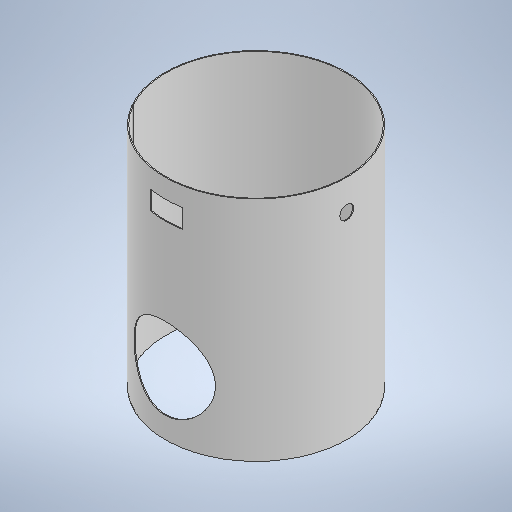
# Autodesk Inventor part: PRS 000 Filter1200 MAIN Shell
Saved by Autodesk Inventor 2026.2 (Build 302298000, 298)
## iProperties
Created: 2025-02-11
Part Number: PRS 000 Filter1200 MAIN Shell
Material: Steel
Document SubType Name: Sheet Metal
Designer: pokla
Mass: 197479 g
Surface Area: 84554.1 cm^2
Volume: 25156.5 cm^3
Density: 7.85 g/cm^3
Flat Pattern Width: 150 cm
Flat Pattern Length: 374.776 cm
Flat Pattern Area: 56216.4 cm^2
Sheet Metal Rule: Default_mm
Sheet Metal Width: 1500,000 mm
Sheet Metal Length: 3747,758 mm
Sheet Metal Area: 5621637,523 mm^2
Appearance: Default
Author: pokla
Autodesk Inventor part; units mm, degrees
sketch "Sketch13" plane through (0, 0, 0) normal (0, 0, 1) x (1, 0, 0)
  circle A0 centre (0, 0) radius 600 construction
  line L0 (0, 0) -> (0, -600)
  line L1 (0, 0) -> (-519.6152, -300)
  line L2 (0, 0) -> (600, 0)
  line L3 (0, 0) -> (0, -600)
  line L4 (0, 0) -> (0, -600)
  line L5 (0, 0) -> (534.6039, 272.3943)
  line L6 (0, 0) -> (0, 600)
  dimension "d53" = 1200
  dimension "d55" = 0
  dimension "d98" = 180
  dimension "d99" = 240
  dimension "d100" = 63
  dimension "d101" = 90
  constraints: 14 end point, 1 coincident, 1 point on line, 1 vertical, 9 other
  measures "d55" distance between parallel lines of L0 L4
  measures "d98" angle of L3 L6
  measures "d100" angle of L6 L5
  measures "d101" angle of L2 L6
ref_plane "WeldJoint" through (0, 0, -10) normal (0.5, -0.866, 0) x (0, 0, 1)
ref_plane "Inlet_Clock_Angle_plane" through (0, 0, -10) normal (0, 1, 0) x (0, 0, 1)
ref_plane "Charging" through (0, 0, -10) normal (1, 0, 0) x (0, 0, 1)
ref_plane "Accsess" through (0, 0, -10) normal (1, 0, 0) x (0, 0, 1)
sketch "Sketch14" plane through (0, 0, -10) normal (0.5, -0.866, 0) x (0, 0, 1)
  line L0 (1510, 594) -> (10, 594)
  line L1 (10, 594) -> (10, 600)
  line L2 (10, 600) -> (1510, 600)
  line L3 (1510, 600) -> (1510, 594)
  line L4 (10, 0) -> (1510, 0)
  line L5 (10, 600) -> (-20, 600) construction
  line L6 (10, 594) -> (-20, 594) construction
  arc A0 (-20, 594) -> (-109.2789, 539.0476) centre (-20, 494) ccw construction
  arc A1 (-109.2789, 539.0476) -> (-234, 15) centre (929.3202, 15) ccw construction
  line L7 (-234, 15) -> (-234, 0) construction
  line L8 (10, 0) -> (-234, 0) construction
  arc A2 (-20, 600) -> (-114.6356, 541.7504) centre (-20, 494) ccw construction
  arc A3 (-114.6356, 541.7504) -> (-240, 15) centre (929.3202, 15) ccw construction
  line L9 (-240, 15) -> (-240, 0) construction
  line L10 (-234, 0) -> (-240, 0) construction
  line L11 (1510, 594) -> (1540, 594)
  line L12 (1510, 600) -> (1540, 600)
  line L13 (1510, 0) -> (1754, 0) construction
  line L14 (1760, 0) -> (1760, 15) construction
  arc A4 (1760, 15) -> (1634.6356, 541.7504) centre (590.6798, 15) ccw construction
  arc A5 (1634.6356, 541.7504) -> (1540, 600) centre (1540, 494) ccw construction
  line L15 (1754, 0) -> (1754, 15) construction
  line L16 (1754, 0) -> (1760, 0) construction
  arc A6 (1754, 15) -> (1629.2789, 539.0476) centre (590.6798, 15) ccw construction
  arc A7 (1629.2789, 539.0476) -> (1540, 594) centre (1540, 494) ccw construction
  line L17 (-156.8588, 530) -> (-610, 530)
  line L18 (-610, 530) -> (-610, 450)
  line L19 (-610, 450) -> (-156.8588, 450)
  line L20 (-156.8588, 450) -> (-156.8588, 530)
  line L21 (1760, 15) -> (1790, 15) construction
  line L22 (1790, 15) -> (1790, 0) construction
  line L23 (1790, 0) -> (1760, 0) construction
  line L24 (-610, 610) -> (-610, 530)
  line L25 (-610, 610) -> (-604, 610)
  line L26 (-604, 610) -> (-604, 530)
  line L27 (-115.4356, 543.7196) -> (-164.9441, 431.7071)
  line L28 (-156.8588, 530) -> (-121.4996, 530)
  line L29 (-109.2789, 539.0476) -> (-114.6356, 541.7504)
  line L30 (-115.4356, 543.7196) -> (-116.0014, 542.4396) construction
  line L31 (-116.0014, 542.4396) -> (-114.6356, 541.7504) construction
  point P0 (10, 597)
  point P1 (-140.1899, 487.7134)
  dimension "d59" = 1500
  dimension "d60" = 6
  dimension "d61" = 1200
  dimension "d82" = 100
  dimension "d83" = 30
  dimension "d86" = 80
  dimension "d87" = 30
  dimension "d88" = 2400
  dimension "d90" = 900
  dimension "d91" = 15
  dimension "d92" = 20
  dimension "d93" = 250
  dimension "d94" = 30
  constraints: 64 end point, 18 point on circle, 13 tangent, 12 horizontal, 8 centre point, 7 perpendicular, 6 equal length, 6 point on line, 4 concentric, 4 parallel, 2 collinear, 2 equal radius, 2 midpoint, 2 vertical, 1 vertical alignment
  measures "d59" distance of L1.end L2.end
  measures "d60" distance of L0.end L1.end
  measures "d61" diameter of L2 L4
  measures "d82" radius of A0
  measures "d83" distance of L0.end L6.end
  measures "d86" distance of L17.end L18.end
  measures "d87" distance of L14.end L21.end
  measures "d88" distance between parallel lines of L22 L18
  measures "d90" diameter of L19 L4
  measures "d91" distance of L28.end L27.start
  measures "d92" distance of L19.end L27.end
  measures "d93" distance of L9.end L4.start
  measures "d94" diameter of L9.start L4
revolve "Revolution2" add sketch "Sketch14" angle 359.9 about axis through (0, 0, 0) along (0, 0, 1) contours L0 L1 L2 L3
sketch "Sketch AnglePlane_InletPipe" plane through (0, 0, -10) normal (0, 1, 0) x (0, 0, 1)
  line L0 (10, -600) -> (10, 600) projected
  line L1 (10, 0) -> (1310, 0)
  line L2 (1310, 0) -> (1310, 600)
  line L3 (1310, 600) -> (10, 600)
  line L4 (10, 600) -> (10, 0)
  point P0 (10, -519.6152)
  point P1 (10, -520.138)
  dimension "d63" = 1200
  dimension "d64" = 90
  dimension "frd_hght" = 1300
  constraints: 8 end point, 1 collinear, 1 horizontal, 1 parallel
  measures "d63" diameter of L3 L1
  measures "d64" angle of L2 L3
  measures "frd_hght" distance of L2.end L3.end
ref_plane "InletPipe_AnglePlane" through (0, 0, 1300) normal (1, 0, 0) x (0, 1, 0)
sketch "Sketch16" plane through (0, 0, 1300) normal (1, 0, 0) x (0, 1, 0)
  circle A0 centre (0, 0) radius 45.5
  point P0 (0, -1300)
  point P1 (0, 0)
  point P2 (0, 0)
  point P3 (0, 0)
  dimension "d66" = 91
  constraints: 1 centre point, 1 coincident
  measures "d66" diameter of A0
extrude "Extrusion7" cut sketch "Sketch16" along normal through all
ref_plane "Work Plane16" through (0, 0, 0) normal (0, -1, 0) x (1, 0, 0)
sketch "Sketch17" plane through (0, 0, 0) normal (0, -1, 0) x (1, 0, 0)
  circle A0 centre (0, 408.5) radius 268.5
  line L0 (0, 140) -> (-495.5727, 140)
  point P0 (0, 0)
  dimension "d69" = 537
  dimension "d71" = 140
  constraints: 2 end point, 2 horizontal, 2 vertical alignment, 2 other
  measures "d71" distance from line of point (0, 0) L0
extrude "Extrusion8" cut sketch "Sketch17" along normal through all
sketch "Sketch19" plane through (0, 0, -10) normal (1, 0, 0) x (0, 0, 1)
  line L0 (10, 0) -> (1260, 0)
  line L1 (1260, 0) -> (1260, 600)
  line L2 (1260, 600) -> (10, 600)
  line L3 (10, 600) -> (10, 0)
  dimension "d74" = 1250
  dimension "d76" = 1200
  dimension "d77" = 90
  constraints: 8 end point, 1 horizontal, 1 parallel, 1 perpendicular
  measures "d74" distance of L1.end L2.end
  measures "d76" diameter of L2 L0
  measures "d77" angle of L2 L1
ref_plane "Work Plane18" through (0, 0, 1250) normal (0, -1, 0) x (1, 0, 0)
sketch "Sketch20" plane through (0, 0, 1250) normal (0, -1, 0) x (1, 0, 0)
  line L0 (-103.5, 0) -> (103.5, 0)
  line L1 (103.5, 0) -> (103.5, 125)
  line L2 (103.5, 125) -> (-103.5, 125)
  line L3 (-103.5, 125) -> (-103.5, 0)
  point P0 (0, -1250)
  point P1 (0, 0)
  point P2 (0, 0)
  point P3 (0, 0)
  point P4 (0, 0)
  dimension "d78" = 207
  dimension "d79" = 125
  constraints: 8 end point, 2 parallel, 1 coincident, 1 horizontal, 1 midpoint, 1 perpendicular
  measures "d78" distance of L2.end L1.end
  measures "d79" distance of L1.end L0.end
extrude "Extrusion9" cut sketch "Sketch20" along normal through all
equation "\"BendRadius\" = Thickness"
equation "\"BendReliefWidth\" = Thickness"
equation "\"BendReliefDepth\" = 0.5 * Thickness"
equation "\"CornerReliefSize\" = 4 * Thickness"
equation "\"MinimumRemnant\" = 2 * Thickness"
equation "\"TransitionRadius\" = BendRadius"
equation "\"JacobiRadiusSize\" = BendRadius"
equation "\"GapSize\" = Thickness"
equation "\"InletPipe_horisont_angle\" = 0"
equation "\"AccsessHatch_diameter\" = 535"
equation "\"AccsessHatch_ClockAngle\" = 0"
equation "\"ChargingHatch_ClockAgnle\" = 180deg"
equation "\"InletPipe_Clock_angle\" = 90deg"
equation "\"OutletPipe_ClockAngle\" = 63deg"
equation "\"WeldJoint_ClockAgnle\" = 240deg"
equation "\"Thickness\" = 6"
body "Solid2"
